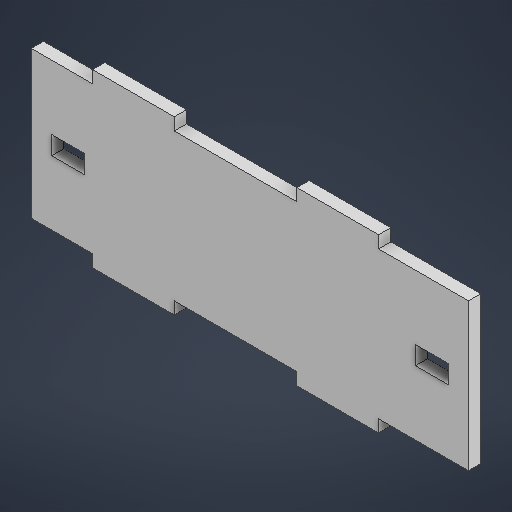
# Autodesk Inventor part: TB6600holder
Saved by Autodesk Inventor 2027 (Build 310192000, 192)
## iProperties
Created: 2026-06-02
Part Number: TB6600holder
Material: Generic
Document SubType Name: Modeling
Designer: alexy
Density: 1 g/cm^3
Appearance: Default
Author: alexy
Autodesk Inventor part; units mm, degrees
ref_plane "YZ Plane" through (0, 0, 0) normal (1, 0, 0) x (0, 1, 0)
ref_plane "XZ Plane" through (0, 0, 0) normal (0, 1, 0) x (-1, 0, 0)
ref_plane "XY Plane" through (0, 0, 0) normal (0, 0, 1) x (1, 0, 0)
sketch "Sketch1" plane through (0, 0, 0) normal (0, 0, 1) x (1, 0, 0)
  line L0 (0, 0) -> (107, 0)
  line L1 (107, 0) -> (107, 36)
  line L2 (107, 36) -> (0, 36)
  line L3 (0, 36) -> (0, 0)
  line L4 (0, 15.75) -> (0, 20.25)
  line L5 (15, 36) -> (35, 36)
  line L6 (35, 36) -> (35, 39)
  line L7 (35, 39) -> (15, 39)
  line L8 (15, 39) -> (15, 36)
  line L9 (65, 36) -> (85, 36)
  line L10 (85, 36) -> (85, 39)
  line L11 (85, 39) -> (65, 39)
  line L12 (65, 39) -> (65, 36)
  line L13 (15, 0) -> (35, 0)
  line L14 (35, 0) -> (35, -3)
  line L15 (35, -3) -> (15, -3)
  line L16 (15, -3) -> (15, 0)
  line L17 (65, 0) -> (85, 0)
  line L18 (85, 0) -> (85, -3)
  line L19 (85, -3) -> (65, -3)
  line L20 (65, -3) -> (65, 0)
  line L21 (5, 20.25) -> (13, 20.25)
  line L22 (13, 20.25) -> (13, 15.75)
  line L23 (13, 15.75) -> (5, 15.75)
  line L24 (5, 15.75) -> (5, 20.25)
  line L25 (94, 20.25) -> (102, 20.25)
  line L26 (102, 20.25) -> (102, 15.75)
  line L27 (102, 15.75) -> (94, 15.75)
  line L28 (94, 15.75) -> (94, 20.25)
  point P0 (102, 18)
  dimension "d0" = 36
  dimension "d1" = 107
  dimension "d6" = 3
  dimension "d7" = 3
  dimension "d8" = 30
  dimension "d9" = 20
  dimension "d10" = 20
  dimension "d11" = 15
  dimension "d14" = 4.5
  dimension "d15" = 8
  dimension "d16" = 8
  dimension "d18" = 97
  dimension "d19" = 5
  dimension "d20" = 18
  constraints: 58 end point, 14 parallel, 10 point on line, 7 horizontal, 7 perpendicular, 4 horizontal alignment, 4 vertical alignment, 1 midpoint
  measures "d0" distance of L0.end L1.end
  measures "d1" distance of L1.end L2.end
  measures "d6" distance of L7.end L5.start
  measures "d7" distance of L15.end L13.start
  measures "d8" distance of L11.end L6.end
  measures "d9" distance of L6.end L7.end
  measures "d10" distance of L10.end L11.end
  measures "d11" horizontal distance of L2.end L7.end
  measures "d14" distance of L25.end L26.end
  measures "d15" distance of L25.start L25.end
  measures "d16" distance of L21.start L21.end
  measures "d18" distance of L23.end L26.end
  measures "d19" distance from line of L1 L26.end
  measures "d20" distance from line of L2 point (102, 18)
extrude "Extrusion1" add sketch "Sketch1" along normal blind 3
body "Solid1"
